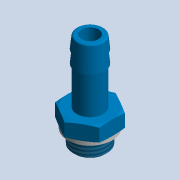
# Autodesk Inventor part: 3607 N-1/4-P-9
Saved by Autodesk Inventor 2021 (Build 250183000, 183)
## iProperties
Category: PARTsolutions
Company: FESTO
Part Number: 3607 N-1/4-P-9
Material: Generic
Catalog Web Link: www.cadenas.de
Description: N-..-P--barbed hose fitting
Vendor: FESTO
Document SubType Name: Modeling
Designer: partserver
Manufacturer: FESTO
Mass: 3.22738 g
Surface Area: 25.9749 cm^2
Volume: 3.22738 cm^3
Density: 1 g/cm^3
Appearance: PSOLRGB-0-145-219
PSOL_IDENT_0: {$CADENAS_DATA\23d-libs\festo\parts\n\n\n_p.prj},169 {VTYP=3D},{NB=3607 N-1/4-P-9},{LINA=3607 N-1/4-
PSOL_IDENT_1: P-9},{NN=N-..-P-},{DATE=27.04.2020 09:06:56},{GEOMDATE=25.09.2015 08:17:00},{VERSION=},{LINEID=30},{
PSOL_IDENT_2: WBVAR=},{WBNUMERIC=}  {NB=3607 N-1/4-P-9},{LINA=3607 N-1/4-P-9},{KT=DUMMY},{TNR=3607},{TYP=N-1/4-P-9
PSOL_IDENT_3: },{L=37.100},{L1=7.000},{L2=24.100},{B=6.000},{D1=G1/4},{D1M=13.157},{D2=10.000},{NENN=6.500},{S=17.
PSOL_IDENT_4: 000},{VER=1}
NB: 3607 N-1/4-P-9
NN: N-..-P-
NT: barbed hose fitting
NBSYN: $TNR. $TYP.
LINA: 3607 N-1/4-P-9
CATALOG: Festo
TNR: 3607
TYP: N-1/4-P-9
L: 37.1
L1: 7
L2: 24.1
B: 6
D1: G1/4
D2: 10
NENN: 6.5
S: 17
SUPPLIER: FESTO
ARTICLENO: 3607 N-1/4-P-9
BOMINFO: 3607 N-1/4-P-9
CREATOR: CADENAS GmbH
Title: 3607 N-1/4-P-9
Author: Cadenas PARTsolutions
Comments: barbed hose fitting
Autodesk Inventor part; units mm, degrees
ref_plane "YZ Plane" through (0, 0, 0) normal (1, 0, 0) x (0, 1, 0)
ref_plane "XZ Plane" through (0, 0, 0) normal (0, 1, 0) x (-1, 0, 0)
ref_plane "XY Plane" through (0, 0, 0) normal (0, 0, 1) x (1, 0, 0)
sketch "Skizze_1" plane through (0, 0, 0) normal (1, 0, 0) x (0, 1, 0)
  line L0 (0, -37.1) -> (0, 0)
  line L1 (0, 0) -> (5.7225, 0)
  line L2 (5.7225, 0) -> (6.5785, -0.856)
  line L3 (6.5785, -0.856) -> (6.5785, -6)
  line L4 (6.5785, -6) -> (8.5, -6)
  line L5 (8.5, -6) -> (8.5, -7.4)
  line L6 (8.5, -7.4) -> (10.2, -7.8555)
  line L7 (10.2, -7.8555) -> (10.2, -12.5445)
  line L8 (10.2, -12.5445) -> (8.5, -13)
  line L9 (8.5, -13) -> (5, -13)
  line L10 (5, -13) -> (5, -27.46)
  line L11 (5, -27.46) -> (5.5, -27.46)
  line L12 (5.5, -27.46) -> (5, -32.28)
  line L13 (5, -32.28) -> (5.5, -32.28)
  line L14 (5.5, -32.28) -> (5.0558, -36.5619)
  arc A0 (4.459, -37.1) -> (5.0558, -36.5619) centre (4.459, -36.5) ccw
  line L15 (4.459, -37.1) -> (0, -37.1)
  line L16 (0, -37.1) -> (0, 0)
  constraints: 34 end point, 2 point on circle, 1 centre point
revolve "Revolution1" add sketch "Skizze_1" angle 360 about axis through (0, 0, -37.1) along (0, 0, -1)
thread "Thread1" size "G13.157x1.337" designation "G 1/4" class "A" standard "ISO Pipe Threads" length 4.144
sketch "Sketch2" plane through (0, 0, 0) normal (0, 0, 1) x (1, 0, 0)
  point P0 (0, 0)
hole "Hole1" at (0, 0, 0) direction (0, 0, -1) diameter 6.5 depth 37.1 countersink diameter 8.8094 countersink angle 60
sketch "Skizze_3" plane through (0, 0, 0) normal (0, 0, 1) x (1, 0, 0)
  line L0 (-17, -17) -> (17, -17)
  line L1 (17, -17) -> (17, 17)
  line L2 (17, 17) -> (-17, 17)
  line L3 (-17, 17) -> (-17, -17)
  line L4 (-8.5, -4.9075) -> (0, -9.815)
  line L5 (0, -9.815) -> (8.5, -4.9075)
  line L6 (8.5, -4.9075) -> (8.5, 4.9075)
  line L7 (8.5, 4.9075) -> (0, 9.815)
  line L8 (0, 9.815) -> (-8.5, 4.9075)
  line L9 (-8.5, 4.9075) -> (-8.5, -4.9075)
  constraints: 20 end point
extrude "Extrusion1" cut sketch "Skizze_3" against normal blind 13
ref_plane "ANBAU_XY" through (0, 0, -6) normal (0, 0, -1) x (1, 0, 0)
ref_plane "ANBAU_YZ" through (0, 0, -6) normal (1, 0, 0) x (0, -1, 0)
ref_plane "ANBAU_ZX" through (0, 0, -6) normal (0, -1, 0) x (0, 0, -1)
ref_plane "ANBAU_STD_XY" through (0, 0, -6) normal (0, 0, -1) x (1, 0, 0)
ref_plane "ANBAU_STD_YZ" through (0, 0, -6) normal (1, 0, 0) x (0, -1, 0)
ref_plane "ANBAU_STD_ZX" through (0, 0, -6) normal (0, -1, 0) x (0, 0, -1)
body "Solid1"
